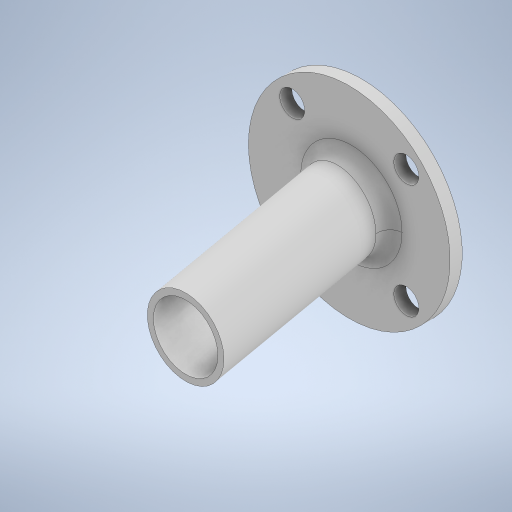
# Autodesk Inventor part: SoporteMarcador
Saved by Autodesk Inventor 2023 (Build 270158000, 158)
## iProperties
Created: 2023-09-03
Part Number: SoporteMarcador
Material: Generic
Document SubType Name: Modeling
Designer: felip
Density: 1 g/cm^3
Appearance: Default
Author: felip
Autodesk Inventor part; units mm, degrees
ref_plane "YZ Plane" through (0, 0, 0) normal (1, 0, 0) x (0, 1, 0)
ref_plane "XZ Plane" through (0, 0, 0) normal (0, 1, 0) x (-1, 0, 0)
ref_plane "XY Plane" through (0, 0, 0) normal (0, 0, 1) x (1, 0, 0)
sketch "Sketch2" plane through (0, 0, 0) normal (0, 0, 1) x (-1, 0, 0)
  circle A0 centre (0, 0) radius 25
  line L0 (0, 0) -> (20, 0) construction
  line L1 (0, 0) -> (20, 0) construction
  line L2 (0, 0) -> (20, 0) construction
  line L3 (0, 0) -> (20, 0) construction
  circle A1 centre (14.1421, 14.1421) radius 3.125
  circle A2 centre (-14.1421, 14.1421) radius 3.125
  circle A3 centre (-14.1421, -14.1421) radius 3.125
  circle A4 centre (14.1421, -14.1421) radius 3.125
  dimension "d0" = 50
  dimension "d10" = 6.25
  dimension "d11" = 6.25
  dimension "d12" = 6.25
  dimension "d13" = 6.25
  constraints: 8 end point, 5 centre point, 4 horizontal, 2 coincident
  measures "d0" diameter of A0
  measures "d10" diameter of A1
  measures "d11" diameter of A2
  measures "d12" diameter of A3
  measures "d13" diameter of A4
extrude "Extrusion1" add sketch "Sketch2" along normal blind 3
sketch "Sketch19" plane through (0, 0, 3) normal (0, 0, 1) x (1, 0, 0)
  circle A0 centre (0, 0) radius 9.5
  dimension "d40" = 19
  constraints: 1 centre point, 1 coincident
  measures "d40" diameter of A0
sketch "Sketch22" plane through (0, 0, 0) normal (0, 1, 0) x (-1, 0, 0)
  line L0 (25, 3) -> (-25, 3) projected
  line L1 (0, 3) -> (-8.6824, 52.2404)
  line L2 (0, 3) -> (50, 3) construction
  point P0 (0, 0)
  dimension "d41" = 50
  dimension "d42" = 100
  constraints: 4 end point, 1 equal length, 1 horizontal, 1 midpoint
  measures "d41" distance of L1.start L1.end
  measures "d42" angle of L2 L1
sweep "Sweep4" add profiles "Sketch19" path "Sketch22" path curves L1
sketch "Sketch23" plane through (0, 0, 3) normal (0, 0, 1) x (1, 0, 0)
  circle A0 centre (0, 0) radius 8
  dimension "d45" = 16
  constraints: 1 centre point, 1 coincident
  measures "d45" diameter of A0
sketch "Sketch25" plane through (0, 0, 0) normal (0, 1, 0) x (-1, 0, 0)
  line L0 (25, 3) -> (-25, 3) projected
  line L1 (0, 3) -> (-8.6824, 52.2404)
  line L2 (0, 3) -> (50, 3) construction
  point P0 (0, 0)
  dimension "d46" = 50
  dimension "d47" = 100
  constraints: 4 end point, 1 equal length, 1 horizontal, 1 midpoint
  measures "d46" distance of L1.start L1.end
  measures "d47" angle of L2 L1
sweep "Sweep5" cut profiles "Sketch23" path "Sketch25" path curves L1
fillet "Fillet2" radius 3 1 edges at (-9.5, 0, 3)
body "Solid1"
